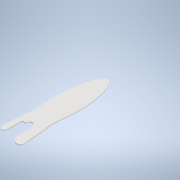
# Autodesk Inventor part: Board
Saved by Autodesk Inventor 2021 (Build 250183000, 183)
## iProperties
Created: 2021-03-08
Part Number: Board
Material: Generic
Document SubType Name: Modeling
Designer: bl17
Density: 1 g/cm^3
Appearance: Default
Author: bl17
Autodesk Inventor part; units mm, degrees
ref_plane "YZ Plane" through (0, 0, 0) normal (1, 0, 0) x (0, 1, 0)
ref_plane "XZ Plane" through (0, 0, 0) normal (0, 1, 0) x (-1, 0, 0)
ref_plane "XY Plane" through (0, 0, 0) normal (0, 0, 1) x (1, 0, 0)
sketch "Sketch2" plane through (0, 0, 0) normal (0, 1, 0) x (-1, 0, 0)
  line L0 (194.6579, -241.6418) -> (-40.2921, -241.6418) construction
  line L1 (-30.7671, -644.5615) -> (185.1329, -644.5615) construction
  line L2 (147.0329, 110.1905) -> (147.0329, 62.5655)
  line L3 (209.9876, 110.1905) -> (-95.098, 110.1905) construction
  arc A0 (147.0329, 62.5655) -> (147.0329, 56.2155) centre (147.0329, 59.3905) ccw
  line L4 (97.2679, -54.9095) -> (57.0979, -54.9095) construction
  line L5 (97.2679, -54.9095) -> (137.4379, -54.9095) construction
  line L6 (77.1829, -834.8709) -> (77.1829, 198.0101) construction
  line L7 (147.0329, 56.2155) -> (147.0329, -16.8095)
  line L8 (147.0329, 62.5655) -> (147.0329, 56.2155) construction
  line L9 (235, 132.4241) -> (-116.3118, 132.4241) construction
  line L10 (235, 132.4241) -> (586.3118, 132.4241) construction
  arc A1 (39.0829, 56.2155) -> (39.0829, 62.5655) centre (39.0829, 59.3905) ccw
  line L11 (39.0829, 62.5655) -> (39.0829, 56.2155) construction
  line L12 (39.0829, 62.5655) -> (45.4329, 62.5655) construction
  line L13 (39.0829, 56.2155) -> (39.0829, -16.8095)
  line L14 (39.0829, 110.1905) -> (39.0829, 62.5655)
  line L15 (107.9631, -23.1595) -> (33.1393, -23.1595) construction
  line L16 (107.9737, -23.1595) -> (107.9631, -23.1595) construction
  arc A2 (45.4329, -23.1595) -> (108.9329, -23.1595) centre (77.1829, -23.1595) ccw
  line L17 (108.9329, -23.1595) -> (45.4329, -23.1595) construction
  line L18 (108.9329, -23.1595) -> (172.4329, -23.1595) construction
  line L19 (147.0329, -16.8095) -> (108.9329, -16.8095)
  line L20 (108.9329, -16.8095) -> (108.9329, -23.1595)
  line L21 (45.4329, -23.1595) -> (45.4329, -16.8095)
  line L22 (45.4329, -23.1595) -> (51.7829, -23.1595) construction
  line L23 (45.4329, -16.8095) -> (39.0829, -16.8095)
  arc A3 (39.0829, 110.1905) -> (-46.6421, 110.1905) centre (-3.7796, 79.9915) ccw
  arc A4 (201.0079, 110.1905) -> (147.0329, 110.1905) centre (174.0204, 104.9283) ccw
  line L24 (191.4829, -84.5811) -> (-37.1171, -84.5811) construction
  line L25 (201.0079, 110.1905) -> (191.4829, -84.5811)
  line L26 (-46.6421, 110.1905) -> (-37.1171, -84.5811)
  spline S0 degree 4 poles (191.4829, -84.5811) (153.3095, -195.3959) (291.7997, -323.3196) (77.1829, -1372.7001) (-137.4339, -323.3196) (1.0563, -195.3959) (-37.1171, -84.5811) knots 0 0 0 0 0 0.408052 0.591948 1 1 1 1 1
  point P0 (77.1829, -241.6418)
  point P1 (77.1829, -779.6686)
  point P2 (5.0659, 158.3555)
  point P3 (77.1829, -644.5615)
  point P4 (77.1829, -36.1166)
  point P5 (77.1829, -54.9095)
  point P6 (77.1829, -84.5811)
  dimension "d20" = 234.95
  dimension "d37" = 215.9
  dimension "d51" = 6.35
  dimension "d52" = 50.8
  dimension "d60" = 180
  dimension "d61" = 114.3
  dimension "d76" = 180
  dimension "d81" = 6.35
  dimension "d82" = 90
  dimension "d83" = 3.175
  dimension "d84" = 50.8
  dimension "d85" = 69.85
  dimension "d86" = 38.1
  dimension "d98" = 63.5
  dimension "d99" = 180
  dimension "d100" = 31.75
  dimension "d101" = 90
  dimension "d102" = 76.2
  dimension "d106" = 247.65
  dimension "d107" = 123.825
  dimension "d108" = 228.6
  constraints: 55 end point, 13 horizontal, 12 point on line, 11 point on circle, 5 centre point, 5 equal length, 5 vertical, 4 midpoint, 2 collinear, 2 perpendicular, 2 tangent, 7 other
  measures "d20" distance of L0.start L0.end
  measures "d37" distance of L1.start L1.end
  measures "d51" diameter of A0
  measures "d52" distance of L2.start A0.centre
  measures "d60" angle of L4 L5
  measures "d61" distance from line of L4 A0.centre
  measures "d76" angle of L9 L10
  measures "d81" distance of L11.start L11.end
  measures "d82" angle of L11 L12
  measures "d83" radius of A1
  measures "d84" distance of L14.start A1.centre
  measures "d85" distance between parallel lines of L6 L2
  measures "d86" distance between parallel lines of L6 L14
  measures "d98" distance of L17.start L17.end
  measures "d99" angle of L17 L18
  measures "d100" radius of A2
  measures "d101" angle of L22 L21
  measures "d102" distance from line of L19 A0.centre
  measures "d106" distance of L25.start L26.start
  measures "d107" distance from line of L6 L26.start
  measures "d108" distance of L24.start L24.end
extrude "Extrusion2" add sketch "Sketch2" along normal blind 9.525
fillet "Fillet2" radius 6.35 1 edges at (-39.0829, 4.7625, -16.8095)
fillet "Fillet3" radius 6.35 2 edges at (-45.4324, 4.7625, -16.8095) (-45.4329, 4.7625, -16.8095)
fillet "Fillet4" radius 6.35 2 edges at (-108.9329, 4.7625, -16.8095) (-147.0329, 4.7625, -16.8095)
body "Solid2"
